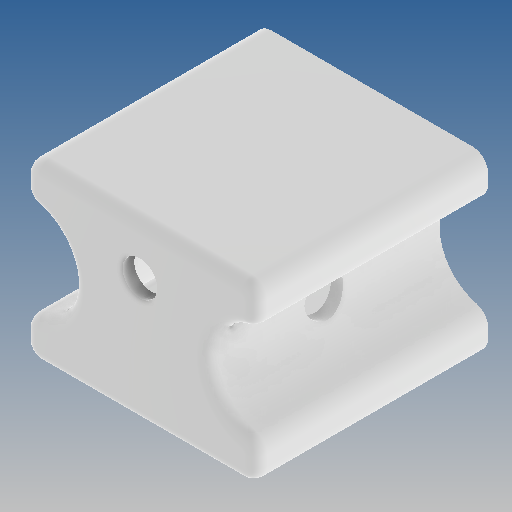
# Autodesk Inventor part: PWTR-0151
Saved by Autodesk Inventor 2021.1 (Build 251245000, 245)
## iProperties
Created: 2020-09-04
Part Number: PWTR-0151
Material: ABS Plastic
Document SubType Name: Modeling
Designer: alid
Density: 1.06 g/cm^3
Appearance: Smooth - White
Description: Lightweight Handle Stretcher
Sheet Metal Rule: Default_mm
Author: alid
Revision Number: A
Autodesk Inventor part; units mm, degrees
ref_plane "YZ Plane" through (0, 0, 0) normal (1, 0, 0) x (0, 1, 0)
ref_plane "XZ Plane" through (0, 0, 0) normal (0, 1, 0) x (-1, 0, 0)
ref_plane "XY Plane" through (0, 0, 0) normal (0, 0, 1) x (1, 0, 0)
sketch "Sketch1" plane through (0, 0, 0) normal (0, 1, 0) x (-1, 0, 0)
  line L0 (0, 22.5) -> (-26, 22.5)
  line L1 (-30, 18.5) -> (-30, 16.0078)
  arc A0 (-26.9697, -12.1271) -> (-26.9697, 12.1271) centre (-30, 0) ccw
  line L2 (-30, -16.0078) -> (-30, -18.5)
  line L3 (-26, -22.5) -> (0, -22.5)
  arc A1 (-26, 22.5) -> (-30, 18.5) centre (-26, 18.5) ccw
  arc A2 (-30, 16.0078) -> (-26.9697, 12.1271) centre (-26, 16.0078) ccw
  arc A3 (-26.9697, -12.1271) -> (-30, -16.0078) centre (-26, -16.0078) ccw
  arc A4 (-30, -18.5) -> (-26, -22.5) centre (-26, -18.5) ccw
  line L4 (0, -22.5) -> (0, 22.5)
  point P0 (-30, 22.5)
  point P1 (-30, 12.5)
  point P2 (-30, -12.5)
  point P3 (-30, -22.5)
  point P4 (0, 0)
  point P5 (0, 0)
  dimension "d2" = 12.5
  dimension "d3" = 10
  dimension "d4" = 10
  dimension "d5" = 4
  dimension "d17" = 45
  dimension "d31" = 30
  constraints: 12 point on circle, 10 end point, 9 point on line, 8 tangent, 5 centre point, 3 equal radius, 2 vertical, 1 coincident, 1 horizontal, 1 midpoint, 1 perpendicular
  measures "d2" radius of A0
  measures "d3" distance of point (-30, 22.5) point (-30, 12.5)
  measures "d4" distance of point (-30, -12.5) point (-30, -22.5)
  measures "d5" radius of A1
  measures "d17" distance between parallel lines of L3 L0
  measures "d31" distance from line of L4 A0.centre
extrude "Extrusion1" add sketch "Sketch1" along normal mid plane 60
mirror "Mirror1" about plane through (0, 0, 0) normal (1, 0, 0)
fillet "Fillet1" radius 3 16 edges at (0, -30, 22.5) (-28.8284, -30, 21.3284) (-30, -30, 17.2539) (-29.1527, -30, 13.546) (-17.5, -30, 0) (-29.1527, -30, -13.546) (-30, -30, -17.2539) (-28.8284, -30, -21.3284) (0, -30, -22.5) (28.8284, -30, -21.3284) (30, -30, -17.2539) (29.1527, -30, -13.546) (17.5, -30, 0) (29.1527, -30, 13.546) (30, -30, 17.2539) (28.8284, -30, 21.3284)
shell "Shell1" thickness 3 removed faces 1 at (6.5675, 30, 17.3619)
sketch "Sketch3" plane through (0, 0, 0) normal (1, 0, 0) x (0, 1, 0)
  circle A0 centre (0, 0) radius 5
  dimension "d32" = 10
  constraints: 1 centre point, 1 coincident
  measures "d32" diameter of A0
extrude "Extrusion2" cut sketch "Sketch3" along normal through all both and the other way through all
sketch "Sketch4" plane through (0, 0, 0) normal (0, 1, 0) x (-1, 0, 0)
  line L0 (0, 0) -> (0, 10)
  dimension "d37" = 10
  constraints: 2 end point, 1 vertical
  measures "d37" distance of L0.start L0.end
hole "Hole1" at (0, 0, 10) direction (0, -1, 0) diameter 9 end through all clearance for "Countersunk Flat Head Screw ISO 2009/7046" size "M8" standard "ISO"
equation "\"d4\" = d3"
equation "\"d5\" = 2 * BendRadius"
equation "\"BendRadius\" = Thickness"
equation "\"BendReliefWidth\" = Thickness"
equation "\"BendReliefDepth\" = 0.5 * Thickness"
equation "\"CornerReliefSize\" = 4 * Thickness"
equation "\"MinimumRemnant\" = 2 * Thickness"
equation "\"TransitionRadius\" = BendRadius"
equation "\"JacobiRadiusSize\" = BendRadius"
equation "\"GapSize\" = Thickness"
equation "\"Thickness\" = 2"
body "Solid1"
body "Solid2"
